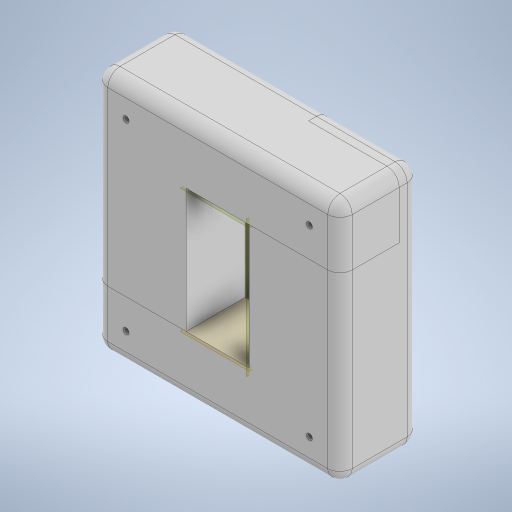
# Autodesk Inventor part: BGO-holder-C-conector
Saved by Autodesk Inventor 2023 (Build 270158000, 158)
## iProperties
Created: 2023-12-01
Part Number: BGO-holder-C-conector
Material: Generic
Document SubType Name: Modeling
Designer: AxLab
Density: 1 g/cm^3
Appearance: Default
Author: AxLab
Autodesk Inventor part; units mm, degrees
ref_plane "YZ Plane" through (0, 0, 0) normal (1, 0, 0) x (0, 1, 0)
ref_plane "XZ Plane" through (0, 0, 0) normal (0, 1, 0) x (-1, 0, 0)
ref_plane "XY Plane" through (0, 0, 0) normal (0, 0, 1) x (1, 0, 0)
sketch "Sketch1" plane through (0, 0, 0) normal (0, 0, 1) x (1, 0, 0)
  line L0 (-20, -20) -> (20, -20)
  line L1 (20, -20) -> (20, 20)
  line L2 (20, 20) -> (-20, 20)
  line L3 (-20, 20) -> (-20, -20)
  line L4 (-20, -20) -> (20, 20) construction
  line L5 (20, -20) -> (-20, 20) construction
  point P0 (0, 0)
  dimension "d0" = 40
  dimension "d1" = 40
  constraints: 12 end point, 2 midpoint, 2 parallel, 1 horizontal, 1 perpendicular
  measures "d0" distance of L2.end L1.end
  measures "d1" distance of L1.end L0.end
extrude "Extrusion1" add sketch "Sketch1" along normal blind 13
sketch "Sketch2" plane through (0, 0, 13) normal (0, 0, 1) x (1, 0, 0)
  line L0 (5.15, -10.15) -> (-5.15, -10.15)
  line L1 (-5.15, -10.15) -> (-5.15, 10.15)
  line L2 (-5.15, 10.15) -> (5.15, 10.15)
  line L3 (5.15, 10.15) -> (5.15, -10.15)
  line L4 (5.15, -10.15) -> (-5.15, 10.15) construction
  line L5 (-5.15, -10.15) -> (5.15, 10.15) construction
  point P0 (0, 0)
  dimension "d4" = 10.3
  dimension "d5" = 20.3
  constraints: 12 end point, 2 midpoint, 2 parallel, 1 horizontal, 1 perpendicular
  measures "d4" distance of L1.end L2.end
  measures "d5" distance of L0.end L1.end
extrude "Extrusion2" cut sketch "Sketch2" against normal blind 9.7
sketch "Sketch3" plane through (0, 0, 13) normal (0, 0, 1) x (1, 0, 0)
  line L0 (-20, 20) -> (-20, -20) projected
  line L1 (-20, 20) -> (-15, 20)
  line L2 (-15, 20) -> (-15, 15)
  line L3 (-15, 15) -> (-20, 15)
  line L4 (-20, 15) -> (-20, 20)
  circle A0 centre (-15, 15) radius 0.5
  point P0 (0, 0)
  dimension "d8" = 5
  dimension "d9" = 5
  dimension "d10" = 1
  constraints: 8 end point, 2 parallel, 1 centre point, 1 coincident, 1 horizontal, 1 perpendicular
  measures "d8" distance of L2.end L3.end
  measures "d9" distance of L1.end L2.end
  measures "d10" diameter of A0
extrude "Extrusion3" cut sketch "Sketch3" against normal blind 13 contours A0 L2 L3 | L3 L2 A0
mirror "Mirror1" about plane through (0, 0, 0) normal (0, 1, 0) of "Extrusion3"
mirror "Mirror2" about plane through (0, 0, 0) normal (1, 0, 0) of "Extrusion3", "Mirror1"
ref_plane "Work Plane1" through (-5.15, -10.15, 13) normal (0, 1, 0) x (1, 0, 0)
ref_plane "Work Plane2" through (-5.15, 10.15, 13) normal (0, -1, 0) x (1, 0, 0)
ref_plane "Work Plane3" through (5.15, -10.15, 13) normal (-1, 0, 0) x (0, 0, 1)
ref_plane "Work Plane4" through (0, 0, 3.3) normal (0, 0, 1) x (1, 0, 0)
split body "Split4" result two bodies by plane through (5.15, -10.15, 13) normal (-1, 0, 0) first body at (-1.4419, -4.8895, 0.5)
split body "Split5" result two bodies by plane through (-5.15, 10.15, 13) normal (0, -1, 0) bodies 3 first body at (13.3632, 1.9321, 0.5)
split body "Split6" result two bodies by plane through (-5.15, -10.15, 13) normal (0, 1, 0) bodies 2 first body at (-9.8909, -1.9225, 0.5)
split body "Split7" result two bodies by plane through (0, 0, 3.3) normal (0, 0, 1) bodies 7 first body at (-4.8524, -15.1275, 3.8)
split body "Split8" result two bodies by plane through (0, 0, 3.3) normal (0, 0, 1) bodies 5 first body at (8.2667, 15.05, 3.8)
combine bodies "Combine1" operation type add bodies to combine 11 4 8
combine bodies "Combine2" operation type add bodies to combine 10 6 9
fillet "Fillet2" radius 2 18 edges at (-20, 20, 6.5) (-20, 0, 0) (-20, -20, 1.65) (-20, 4.925, 13) (0, 20, 13) (-7.425, 20, 0) (20, 15.075, 13) (20, 20, 8.15) (-7.425, -20, 0) (-20, -20, 8.15) (0, -20, 13) (-20, -15.075, 13) (20, -4.925, 13) (20, -20, 6.5) (12.575, 20, 0) (20, 20, 1.65) (20, 0, 0) (12.575, -20, 0)
body "Solid10"
body "Solid11"
